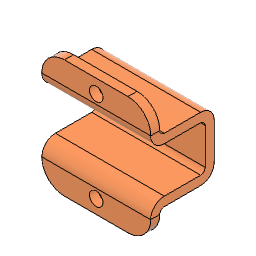
Rover-v23 (Autodesk Fusion 360 archive; units mm, degrees)
design "N20Mount"
Autodesk Fusion 360 part; units mm, degrees
sketch "Profile" plane through (0, 0, 0) normal (1, 0, 0) x (0, 0, -1)
  line L0 (0, 26) -> (0, 21)
  line L1 (3, 18) -> (11, 18)
  line L2 (12, 17) -> (12, 9)
  line L3 (11, 8) -> (3, 8)
  line L4 (0, 5) -> (0, 0)
  arc A0 (12, 17) -> (11, 18) centre (11, 17) ccw
  arc A1 (11, 8) -> (12, 9) centre (11, 9) ccw
  arc A2 (0, 21) -> (3, 18) centre (3, 21) ccw
  arc A3 (3, 8) -> (0, 5) centre (3, 5) ccw
  line L5 (2, 26) -> (2, 21)
  arc A4 (2, 21) -> (3, 20) centre (3, 21) ccw
  line L6 (3, 20) -> (11, 20)
  arc A5 (14, 17) -> (11, 20) centre (11, 17) ccw
  line L7 (14, 17) -> (14, 9)
  arc A6 (11, 6) -> (14, 9) centre (11, 9) ccw
  line L8 (11, 6) -> (3, 6)
  arc A7 (3, 6) -> (2, 5) centre (3, 5) ccw
  line L9 (2, 5) -> (2, 0)
  line L10 (0, 26) -> (2, 26)
  line L11 (0, 0) -> (2, 0)
  point P0 (0, 18)
  point P1 (12, 18)
  point P2 (12, 8)
  point P3 (0, 8)
  point P4 (0, 26)
  dimension "d60" = 10
  dimension "d61" = 12
  dimension "d63" = 8
  dimension "d66" = 1
  dimension "d67" = 3
  dimension "d68" = -2
  constraint vertical L0
  constraint perpendicular L0 L1
  constraint perpendicular L1 L2
  constraint perpendicular L2 L3
  constraint perpendicular L3 L4
  constraint collinear L0 L4
  constraint coincident P1 L1
  constraint coincident P1 L2
  constraint tangent L1 A0
  constraint tangent L2 A0
  constraint coincident P2 L2
  constraint coincident P2 L3
  constraint tangent L2 A1
  constraint tangent L3 A1
  constraint equal A0 A1
  constraint coincident P0 L0
  constraint coincident P0 L1
  constraint tangent L0 A2
  constraint tangent L1 A2
  constraint coincident P3 L3
  constraint coincident P3 L4
  constraint tangent L3 A3
  constraint tangent L4 A3
  constraint equal A2 A3
  constraint equal L0 L4
  constraint coincident P4 L0.start
  constraint coincident L4.end L11.start
  measures "d60" distance of P1 P2
  measures "d61" distance of P0 P1
  measures "d63" distance of P3 L4.end
  measures "d66" radius of A0
  measures "d67" radius of A2
extrude "Extrude1" add sketch "Profile" along normal blind 24
sketch "Sketch5" plane through (0, 0, 0) normal (0, 0, 1) x (1, 0, 0)
  line L0 (0, 5) -> (0, 0)
  line L1 (0, 0) -> (24, 0)
  line L2 (24, 0) -> (24, 5)
  line L3 (24, 5) -> (0, 5)
  line L4 (0, 26) -> (24, 26) construction
  line L5 (12, 0) -> (12, 26) construction
  line L6 (24, 17, -12) -> (24, 9, -12) construction
  line L7 (0, 17, -12) -> (0, 9, -12) construction
  circle A0 centre (12, 3) radius 1.5
  circle A1 centre (12, 23) radius 1.5
  arc A2 (5, 26) -> (0, 21) centre (5, 21) ccw
  arc A3 (24, 21) -> (19, 26) centre (19, 21) ccw
  arc A4 (19, 0) -> (24, 5) centre (19, 5) ccw
  arc A5 (0, 5) -> (5, 0) centre (5, 5) ccw
  line L8 (0, 21) -> (0, 26)
  line L9 (5, 26) -> (0, 26)
  line L10 (19, 26) -> (24, 26)
  line L11 (24, 26) -> (24, 21)
  line L12 (24, 5) -> (24, 0)
  line L13 (24, 0) -> (19, 0)
  line L14 (5, 0) -> (0, 0)
  line L15 (0, 0) -> (0, 5)
  dimension "d72" = 3
  dimension "d73" = 3
  dimension "d74" = 3
  dimension "d77" = 5
  constraint midpoint L1 L5.start
  constraint midpoint L4 L5.end
  constraint coincident L5 A0.centre
  constraint coincident L5 A1.centre
  constraint equal A0 A1
  constraint equal A2 A3
  constraint equal A2 A4
  constraint equal A2 A5
  constraint coincident L4.start L8.end
  constraint tangent A2 L8
  constraint tangent A2 L9
  constraint coincident L4.end L10.end
  constraint tangent A3 L10
  constraint tangent A3 L11
  constraint coincident L1.end L2.start
  constraint tangent A4 L12
  constraint tangent A4 L13
  constraint coincident L0.end L1.start
  constraint tangent A5 L14
  constraint tangent A5 L15
  constraint horizontal L9
  constraint horizontal L10
  constraint horizontal L14
  constraint horizontal L13
  constraint vertical L8
  constraint vertical L11
  constraint vertical L12
  constraint vertical L15
  measures "d72" diameter of A0
  measures "d73" distance of L5.start A0.centre
  measures "d74" distance of L5.end A1.centre
  measures "d77" radius of A2
extrude "Extrude2" cut sketch "Sketch5" against normal blind 2 contours L0 L1 A5 L14 L15 | L1 L2 A4 L12 L13 | A0 | A1 | A2 L8 L9 | A3 L10 L11
equation "d60 = N20Thickness"
equation "d61 = N20Width"
equation "d63 = N20MountFlange"
equation "d66 = N20MountInsideCorner"
equation "d67 = N20MountOutsideCorner"
equation "d68 = -N20MountThicketness"
equation "d69 = N20Length"
equation "d72 = M3Hole"
equation "d73 = ( N20MountFlange - N20MountThicketness ) / 2"
equation "d74 = ( N20MountFlange - N20MountThicketness ) / 2"
equation "d75 = -N20MountThicketness"
equation "ROVER_WIDTH = 80 mm"
equation "M3Hole = 3 mm"
equation "N20Thickness = 10 mm"
equation "N20Length = 24 mm"
equation "N20Width = 12 mm"
equation "N20MountThicketness = 2 mm"
equation "N20MountFlange = 6 mm + N20MountThicketness"
equation "N20MountInsideCorner = 1 mm"
equation "N20MountOutsideCorner = N20MountInsideCorner + N20MountThicketness"
named bodies: "N20Mount"
